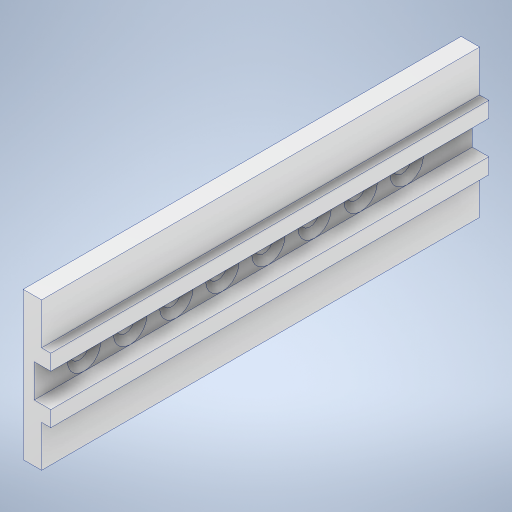
# Autodesk Inventor part: MainRails
Saved by Autodesk Inventor 2024 (Build 280153000, 153)
## iProperties
Created: 2023-08-20
Part Number: MainRails
Material: Aluminum 6061
Document SubType Name: Modeling
Designer: KirikDK
Mass: 3062.81 g
Surface Area: 1947.42 cm^2
Volume: 1134.37 cm^3
Density: 2.7 g/cm^3
Appearance: Aluminum - Flat
Author: KirikDK
Autodesk Inventor part; units mm, degrees
ref_plane "YZ Plane" through (0, 0, 0) normal (1, 0, 0) x (0, 1, 0)
ref_plane "XZ Plane" through (0, 0, 0) normal (0, 1, 0) x (-1, 0, 0)
ref_plane "XY Plane" through (0, 0, 0) normal (0, 0, 1) x (1, 0, 0)
sketch "Sketch1" plane through (0, 0, 0) normal (0, 1, 0) x (-1, 0, 0)
  line L0 (0, 279.3478) -> (-39.1304, 279.3478)
  line L1 (-39.1304, 279.3478) -> (-39.1304, -195.6522)
  line L2 (-39.1304, -195.6522) -> (0, -195.6522)
  line L3 (0, -195.6522) -> (0, 279.3478)
  line L4 (-39.1304, 279.3478) -> (-29.1304, 279.3478)
  line L5 (-29.1304, 254.3478) -> (-39.1304, 254.3478)
  line L6 (-39.1304, 254.3478) -> (-39.1304, 279.3478)
  line L7 (-39.1304, -195.6522) -> (-29.1304, -195.6522)
  line L8 (-29.1304, -170.6522) -> (-39.1304, -170.6522)
  line L9 (-39.1304, -170.6522) -> (-39.1304, -195.6522)
  point P0 (0, 0)
  point P1 (-39.1304, 254.3478)
  dimension "d0" = 475
  dimension "d4" = 25
  dimension "d5" = 25
  dimension "d28" = 39.1304
  constraints: 20 end point, 4 parallel, 3 horizontal, 1 perpendicular
  measures "d0" distance of L2.end L0.start
  measures "d4" distance between parallel lines of L0 L5
  measures "d5" distance between parallel lines of L2 L8
  measures "d28" distance of L0.start L0.end
extrude "Extrusion1" add sketch "Sketch1" along normal blind 160
sketch "Sketch2" plane through (0, 0, 279.3478) normal (0, 0, 1) x (1, 0, 0)
  line L0 (0, 160) -> (39.1304, 160) projected
  line L1 (0, 160) -> (39.1304, 160)
  line L2 (39.1304, 160) -> (39.1304, 0)
  line L3 (39.1304, 0) -> (0, 0)
  line L4 (0, 0) -> (0, 160)
  line L5 (39.1304, 160) -> (29.1304, 160)
  line L6 (29.1304, 160) -> (29.1304, 115)
  line L7 (29.1304, 115) -> (39.1304, 115)
  line L8 (39.1304, 115) -> (39.1304, 160)
  line L9 (39.1304, 0) -> (29.1304, 0)
  line L10 (29.1304, 0) -> (29.1304, 45)
  line L11 (29.1304, 45) -> (39.1304, 45)
  line L12 (39.1304, 45) -> (39.1304, 0)
  circle A0 centre (39.1304, 80) radius 18
  line L13 (21.1304, 75) -> (39.1304, 75)
  line L14 (39.1304, 75) -> (39.1304, 98)
  line L15 (39.1304, 98) -> (21.1304, 98)
  line L16 (21.1304, 98) -> (21.1304, 75)
  line L17 (21.1304, 75) -> (39.1304, 75)
  line L18 (39.1304, 75) -> (39.1304, 62)
  line L19 (39.1304, 62) -> (21.1304, 62)
  line L20 (21.1304, 62) -> (21.1304, 75)
  line L21 (39.1304, 0) -> (39.1304, 160) projected
  line L22 (0, 160) -> (9.1304, 160)
  line L23 (9.1304, 160) -> (9.1304, 0)
  line L24 (9.1304, 0) -> (0, 0)
  line L25 (0, 0) -> (0, 160)
  point P0 (0, 0)
  point P1 (34.1304, 115)
  point P2 (34.1304, 160)
  point P3 (39.1304, 45)
  point P4 (39.1304, 115)
  dimension "d6" = 10
  dimension "d7" = 45
  dimension "d8" = 45
  dimension "d9" = 18
  dimension "d10" = 36
  dimension "d11" = 80
  dimension "d12" = 80
  dimension "d15" = 30
  constraints: 48 end point, 12 parallel, 6 horizontal, 6 perpendicular, 4 point on line, 3 midpoint, 2 point on circle, 1 centre point, 3 other
  measures "d6" distance between parallel lines of L2 L10
  measures "d7" distance between parallel lines of L11 L3
  measures "d8" distance from line of L0 point (34.13, 115)
  measures "d9" distance between parallel lines of L2 L16
  measures "d10" diameter of A0
  measures "d11" distance from line of L3 point (39.13, 80)
  measures "d12" vertical distance of point (34.13, 160) point (39.13, 80)
  measures "d15" distance between parallel lines of L2 L23
extrude "Extrusion2" cut sketch "Sketch2" against normal up to surface (475 mm away) contours L0 L23 L3 L4 | L0 L2 L7 L6 | L10 L11 L2 L3 | L2 L13 A0 | A0 L16 L15 | L2 A0 L13 | A0 L13 L16 | L19 L20 L13 A0
sketch "Sketch3" plane through (21.1304, 62, 279.3478) normal (1, 0, 0) x (0, 0, -1)
  line L0 (475, 0) -> (0, 0) projected
  line L1 (0, 0) -> (0, 36) projected
  line L2 (0, 36) -> (475, 36) projected
  circle A0 centre (54, 18) radius 10
  circle A1 centre (104, 18) radius 10
  circle A2 centre (154, 18) radius 10
  circle A3 centre (204, 18) radius 10
  circle A4 centre (254, 18) radius 10
  circle A5 centre (304, 18) radius 10
  circle A6 centre (354, 18) radius 10
  circle A7 centre (404, 18) radius 10
  circle A8 centre (454, 18) radius 10
  point P0 (279.3478, -62)
  dimension "d18" = 50
  constraints: 9 centre point, 1 horizontal, 16 other
  measures "d18" distance of A0.centre A1.centre
extrude "Extrusion3" cut sketch "Sketch3" against normal blind 25 contours A0 | A1 | A2 | A3 | A4 | A5 | A6 | A7
chamfer "Chamfer1" distance 8 distance2 5 8 edges at (21.1304, 80, 235.3478) (21.1304, 80, 185.3478) (21.1304, 80, 135.3478) (21.1304, 80, 85.3478) (21.1304, 80, 35.3478) (21.1304, 80, -14.6522) (21.1304, 80, -64.6522) (21.1304, 80, -114.6522) measured on face at (21.1304, 80, -64.1522) measured on face at (21.1304, 80, 135.8478) measured on face at (21.1304, 80, 35.8478) measured on face at (21.1304, 80, 185.8478) measured on face at (21.1304, 80, -114.1522) measured on face at (21.1304, 80, -14.1522) measured on face at (21.1304, 80, 85.8478) measured on face at (21.1304, 80, 235.8478)
body "Solid1"
